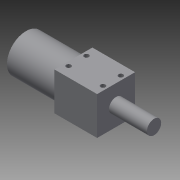
# Autodesk Inventor part: P60 Gear Box
Saved by Autodesk Inventor 2015 (Build 190159000, 159)
## iProperties
Created: 2015-01-11
Part Number: P60 Gear Box
Material: Generic
Document SubType Name: Modeling
Designer: chapale16
Density: 1 g/cm^3
Appearance: Default
Author: chapale16
Autodesk Inventor part; units mm, degrees
ref_plane "YZ Plane" through (0, 0, 0) normal (1, 0, 0) x (0, 1, 0)
ref_plane "XZ Plane" through (0, 0, 0) normal (0, 1, 0) x (-1, 0, 0)
ref_plane "XY Plane" through (0, 0, 0) normal (0, 0, 1) x (1, 0, 0)
sketch "Sketch1" plane through (0, 0, 0) normal (0, 1, 0) x (-1, 0, 0)
  line L0 (41.275, 29.845) -> (-4.445, 29.845)
  line L1 (-4.445, 29.845) -> (-4.445, -10.795)
  line L2 (-4.445, -10.795) -> (41.275, -10.795)
  line L3 (41.275, -10.795) -> (41.275, 29.845)
  circle A0 centre (36.83, 19.05) radius 2.54
  circle A1 centre (36.83, 0) radius 2.54
  circle A2 centre (0, 0) radius 2.54
  circle A3 centre (0, 19.05) radius 2.54
  dimension "d1" = 19.05
  dimension "d2" = 36.83
  dimension "d20" = 40.64
  dimension "d21" = 45.72
  dimension "d22" = 10.795
  dimension "d23" = 4.445
  dimension "d24" = 19.05
  dimension "d25" = 10.795
  dimension "d26" = 36.83
  dimension "d27" = 4.445
  dimension "d28" = 4.445
  dimension "d31" = 5.08
  dimension "d32" = 5.08
  dimension "d33" = 5.08
  dimension "d34" = 5.08
  constraints: 8 end point, 4 centre point, 3 perpendicular, 2 coincident, 1 horizontal
  measures "d1" distance of point (0, 0) point (0, 19.05)
  measures "d2" distance of point (0, 19.05) point (36.83, 19.05)
  measures "d20" distance of L2.end L0.start
  measures "d21" distance of L1.end L2.end
  measures "d22" distance from line of L0 point (36.83, 19.05)
  measures "d23" distance from line of L3 point (36.83, 19.05)
  measures "d24" distance of point (36.83, 0) point (36.83, 19.05)
  measures "d25" distance from line of L0 point (0, 19.05)
  measures "d26" distance of point (36.83, 0) point (0, 0)
  measures "d27" distance from line of L3 point (36.83, 0)
  measures "d28" distance from line of L1 point (0, 0)
  measures "d31" diameter of A0
  measures "d32" diameter of A1
  measures "d33" diameter of A2
  measures "d34" diameter of A3
extrude "Extrusion5" add sketch "Sketch1" along normal blind 40.64
sketch "Sketch4" plane through (0, 40.64, 0) normal (0, 1, 0) x (1, 0, 0)
  point P0 (0, 0)
  point P1 (-18.4878, -9.5896)
sketch "Sketch5" plane through (4.445, 0, 29.845) normal (1, 0, 0) x (0, 0, -1)
  line L0 (0, 40.64) -> (40.64, 0)
  line L1 (40.64, 40.64) -> (0, 0)
  circle A0 centre (20.32, 20.32) radius 7.62
  point P0 (29.845, 0)
  dimension "d38" = 15.24
  constraints: 4 end point, 1 centre point, 1 midpoint
  measures "d38" diameter of A0
extrude "Extrusion6" add sketch "Sketch5" along normal blind 40.64
sketch "Sketch6" plane through (-41.275, 0, -10.795) normal (-1, 0, 0) x (0, 0, 1)
  line L0 (0, 40.64) -> (40.64, 0)
  line L1 (40.64, 40.64) -> (0, 0)
  circle A0 centre (20.32, 20.32) radius 20.32
  point P0 (10.795, 0)
  dimension "d41" = 40.64
  constraints: 4 end point, 1 centre point, 1 midpoint
  measures "d41" diameter of A0
extrude "Extrusion7" add sketch "Sketch6" along normal blind 50.8
body "Solid1"
